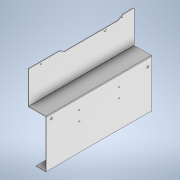
# Autodesk Inventor part: Chapon
Saved by Autodesk Inventor 2020 (Build 240168000, 168)
## iProperties
Created: 2020-06-03
Part Number: Chapon
Material: Aluminum 1100-H14
Document SubType Name: Modeling
Designer: Dante
Density: 2.7 g/cm^3
Appearance: Satin
Author: Dante
Autodesk Inventor part; units mm, degrees
note: some values were not read from the file. Chosen so that the rebuilt part matches the saved one: bend side of "Pieza de plegado4".
ref_plane "YZ Plane" through (0, 0, 0) normal (1, 0, 0) x (0, 1, 0)
ref_plane "XZ Plane" through (0, 0, 0) normal (0, 1, 0) x (-1, 0, 0)
ref_plane "XY Plane" through (0, 0, 0) normal (0, 0, 1) x (1, 0, 0)
sketch "Boceto10" plane through (0, 0, 0) normal (0, 1, 0) x (-1, 0, 0)
  line L0 (9.2786, 29.6594) -> (9.2786, -404.3406)
  line L1 (9.2786, -404.3406) -> (-105.7214, -404.3406)
  line L2 (-105.7214, -404.3406) -> (-105.7214, 29.6594)
  line L3 (-105.7214, 29.6594) -> (9.2786, 29.6594)
  line L4 (-105.7214, 29.6594) -> (-123.7214, 29.6594)
  line L5 (-123.7214, -404.3406) -> (-105.7214, -404.3406)
  line L6 (9.2786, 29.6594) -> (79.7636, 29.6594)
  line L7 (79.7636, 29.6594) -> (79.7636, -404.3406)
  line L8 (79.7636, -404.3406) -> (9.2786, -404.3406)
  line L9 (-123.7214, 29.6594) -> (-123.7214, -98.0201)
  line L10 (-111.7214, -118.8047) -> (-111.7214, -338.8047)
  line L11 (-123.7214, 29.6594) -> (-123.7214, -98.0201)
  line L12 (-123.7214, -359.5893) -> (-123.7214, -404.3406)
  circle A0 centre (-115.7214, -20.3406) radius 2
  circle A1 centre (-115.7214, -354.3406) radius 2
  line L13 (-111.7214, -118.8047) -> (-123.7214, -98.0201)
  line L14 (-111.7214, -338.8047) -> (-123.7214, -359.5893)
  point P0 (0, 0)
  dimension "d65" = 434
  dimension "d66" = 115
  dimension "d67" = 18
  dimension "d76" = 70.485
  dimension "d77" = 434
  dimension "d108" = 220
  dimension "d125" = 4
  dimension "d126" = 8
  dimension "d127" = 50
  dimension "d128" = 4
  dimension "d129" = 8
  dimension "d130" = 50
  dimension "d133" = 18
  dimension "d166" = 12
  constraints: 30 end point, 7 perpendicular, 2 centre point, 2 point on line, 1 horizontal, 1 vertical
  measures "d65" distance of L0.start L0.end
  measures "d66" distance of L0.end L1.end
  measures "d67" distance of L2.end L4.end
  measures "d76" distance of L0.start L6.end
  measures "d77" distance of L6.end L7.end
  measures "d108" distance of L10.start L10.end
  measures "d125" diameter of A0
  measures "d126" distance from line of L9 A0.centre
  measures "d127" distance from line of L4 A0.centre
  measures "d128" diameter of A1
  measures "d129" distance from line of L12 A1.centre
  measures "d130" distance from line of L5 A1.centre
  measures "d133" distance between parallel lines of L12 L2
  measures "d166" distance between parallel lines of L9 L10
extrude "Extrusión13" add sketch "Boceto10" along normal blind 2 contours L0 L1 L2 L3
extrude "Extrusión14" add sketch "Boceto10" along normal blind 2 contours L2 L5 L12 L14 L10 L13 L9 L4
extrude "Extrusión15" add sketch "Boceto10" along normal blind 2 contours L6 L7 L8 L0
bend part "Pieza de plegado2" radius 0.5 angle 90 line through (-9.2786, 0, 29.6594) along (0, 0, -1) centre toward (0, -1, 0) moving side (-1, 0, 0) both sides no
sketch "Boceto11" plane through (-11.7786, -70.1996, -404.3406) normal (-1, 0, 0) x (0, 0, 1)
  line L0 (0, 0) -> (434, 0) projected
  line L1 (434, 0) -> (434, -194.998)
  line L2 (434, -194.998) -> (0, -194.998)
  line L3 (0, -194.998) -> (0, 0)
  circle A0 centre (17, -30) radius 4
  circle A1 centre (414, -15) radius 5
  point P0 (404.3406, 70.1996)
  dimension "d82" = 194.998
  dimension "d158" = 8
  dimension "d159" = 10
  dimension "d161" = 17
  dimension "d162" = 20
  dimension "d164" = 15
  dimension "d165" = 30
  constraints: 6 end point, 2 centre point, 2 perpendicular, 1 vertical
  measures "d82" distance of L0.end L1.end
  measures "d158" diameter of A0
  measures "d159" diameter of A1
  measures "d161" distance from line of A0.centre L3
  measures "d162" distance from line of L1 A1.centre
  measures "d164" distance from line of L0 A1.centre
  measures "d165" distance from line of L0 A0.centre
extrude "Extrusión16" add sketch "Boceto11" against normal blind 2
bend part "Pieza de plegado3" radius 0.5 angle 90 line through (-11.7786, -70.1996, -404.3406) along (0, 0, 1) centre toward (-1, 0, 0) moving side (0, -1, 0) both sides no
sketch "Boceto14" plane through (-206.4912, -70.6996, -404.3406) normal (0, 1, 0) x (1, 0, 0)
  line L0 (0, 0) -> (0, -434) projected
  line L1 (0, -434) -> (-40, -434)
  line L2 (-40, -434) -> (-40, 0)
  line L3 (-40, 0) -> (0, 0)
  line L4 (0, -434) -> (194.2126, -434) projected
  line L5 (194.2126, 0) -> (0, 0) projected
  line L6 (0, -434) -> (0, 0)
  point P0 (206.4912, -404.3406)
  dimension "d91" = 40
  dimension "d92" = 434
  constraints: 8 end point, 1 horizontal, 1 perpendicular, 1 vertical
  measures "d91" distance of L0.end L1.end
  measures "d92" distance of L1.end L2.end
extrude "Extrusión17" add sketch "Boceto14" against normal blind 2
bend part "Pieza de plegado4" radius 0.5 angle 90 line through (-206.4912, -70.6996, -404.3406) along (0, 0, 1) centre toward (0, 1, 0) moving side (1, 0, 0) both sides no
sketch "Boceto15" plane through (-246.4912, -72.6996, 29.6594) normal (0, -1, 0) x (1, 0, 0)
  line L0 (0, -434) -> (0, 0) projected
  line L1 (0, -434) -> (8.8, -434)
  line L2 (-29.6996, -434) -> (40, -434) projected
  circle A0 centre (10, -334) radius 2
  circle A1 centre (10, -100) radius 2
  point P0 (246.4912, -29.6594)
  dimension "d97" = 8.8
  dimension "d98" = 4
  dimension "d99" = 4
  dimension "d101" = 234
  dimension "d102" = 10
  dimension "d103" = 10
  dimension "d136" = 100
  constraints: 2 centre point, 2 end point, 1 point on line
  measures "d97" distance of L0.start L1.end
  measures "d98" diameter of A0
  measures "d99" diameter of A1
  measures "d101" distance of A1.centre A0.centre
  measures "d102" distance from line of L0 A0.centre
  measures "d103" distance from line of L0 A1.centre
  measures "d136" distance from line of L2 A0.centre
extrude "Extrusión18" cut sketch "Boceto15" against normal blind 10
sketch "Boceto16" plane through (-205.9912, -70.1996, 29.6594) normal (-1, 0, 0) x (0, 0, 1)
  circle A0 centre (-135, 111.4272) radius 2
  circle A1 centre (-299, 111.4272) radius 2
  line L0 (0, 193.4272) -> (-434, 193.4272) projected
  line L1 (0, 0) -> (0, 193.4272) projected
  line L2 (-434, 193.4272) -> (-434, 0) projected
  circle A2 centre (-135, 151.4272) radius 2
  circle A3 centre (-299, 151.4272) radius 2
  dimension "d109" = 4
  dimension "d111" = 4
  dimension "d113" = 82
  dimension "d114" = 135
  dimension "d116" = 82
  dimension "d117" = 135
  dimension "d137" = 4
  dimension "d138" = 40
  dimension "d139" = 4
  dimension "d140" = 40
  constraints: 4 centre point
  measures "d109" diameter of A0
  measures "d111" diameter of A1
  measures "d113" distance from line of L0 A0.centre
  measures "d114" distance from line of L1 A0.centre
  measures "d116" distance from line of A1.centre L0
  measures "d117" distance from line of L2 A1.centre
  measures "d137" diameter of A2
  measures "d138" distance of A0.centre A2.centre
  measures "d139" diameter of A3
  measures "d140" distance of A1.centre A3.centre
extrude "Extrusión19" cut sketch "Boceto16" against normal blind 10
sketch "Boceto17" plane through (-278.6908, 126.2276, 29.6594) normal (-1, 0, 0) x (0, 0, 1)
  line L0 (0, 0) -> (0, 133) projected
  line L1 (0, 133) -> (-127.6795, 133) projected
  circle A0 centre (-319, 114.1) radius 1.5
  circle A1 centre (-310, 114.1) radius 1.5
  line L2 (-434, 133) -> (-434, 0) projected
  line L3 (-389.2487, 133) -> (-434, 133) projected
  circle A2 centre (-314.5, 109.5) radius 1.75
  point P0 (-29.6594, -126.2276)
  dimension "d148" = 3
  dimension "d149" = 3
  dimension "d150" = 115
  dimension "d151" = 18.9
  dimension "d152" = 9
  dimension "d153" = 18.9
  dimension "d154" = 3.5
  dimension "d156" = 4.6
  dimension "d157" = 4.5
  constraints: 3 centre point
  measures "d148" diameter of A0
  measures "d149" diameter of A1
  measures "d150" distance from line of L2 A0.centre
  measures "d151" distance from line of L3 A0.centre
  measures "d152" distance of A0.centre A1.centre
  measures "d153" distance from line of L3 A1.centre
  measures "d154" diameter of A2
  measures "d156" vertical distance of A2.centre A1.centre
  measures "d157" horizontal distance of A0.centre A2.centre
extrude "Extrusión20" cut sketch "Boceto17" against normal blind 10
equation "\"d67\" = d133"
equation "\"d126\" = d129"
equation "\"d102\" = d103"
equation "\"d116\" = d113"
equation "\"d153\" = d151"
